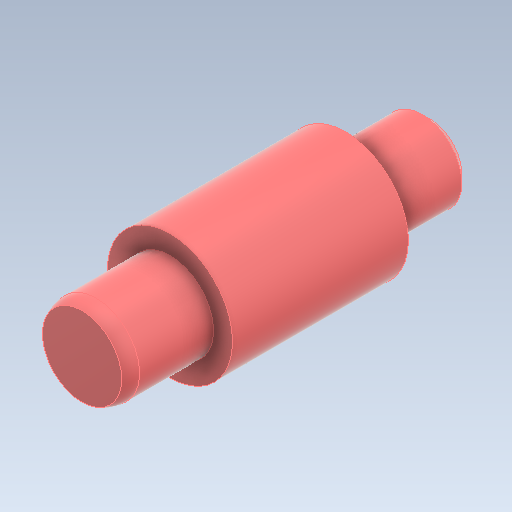
# Autodesk Inventor part: shaft
Saved by Autodesk Inventor 2021 (Build 250183000, 183)
## iProperties
Created: 2022-04-30
Part Number: shaft
Material: Generic
Document SubType Name: Modeling
Designer: authe
Density: 1 g/cm^3
Appearance: Smooth - Red
Author: authe
Autodesk Inventor part; units mm, degrees
ref_plane "YZ Plane" through (0, 0, 0) normal (1, 0, 0) x (0, 1, 0)
ref_plane "XZ Plane" through (0, 0, 0) normal (0, 1, 0) x (-1, 0, 0)
ref_plane "XY Plane" through (0, 0, 0) normal (0, 0, 1) x (1, 0, 0)
sketch "Sketch1" plane through (0, 0, 0) normal (1, 0, 0) x (0, 1, 0)
  line L0 (30.4706, 7.3849) -> (30.4706, 41.1619)
  line L1 (25.6011, 41.1619) -> (24.6173, 41.1619)
  line L2 (25.6011, 62.6619) -> (25.6011, 41.1619)
  line L3 (14.4706, 63.6457) -> (24.6173, 63.6457)
  line L4 (25.6011, 62.6619) -> (24.6173, 63.6457)
  line L5 (25.6011, -3.8381) -> (24.6173, -3.8381)
  line L6 (30.4706, 7.3849) -> (30.4706, -3.8381)
  line L7 (30.4706, 41.1619) -> (25.6011, 41.1619)
  line L8 (30.4706, -3.8381) -> (25.6011, -3.8381)
  line L9 (14.4706, 71.7924) -> (14.4706, 14.0111)
  line L10 (24.6173, -3.8381) -> (24.6173, -23.3381)
  line L11 (22.6173, -25.3381) -> (14.4706, -25.3381)
  line L12 (14.4706, -25.3381) -> (14.4706, 14.0111)
  line L13 (24.6173, -23.3381) -> (22.6173, -25.3381)
  point P0 (24.6173, -25.3381)
  point P1 (14.4706, 63.6457)
  dimension "d26" = 45
  dimension "d27" = 21.5
  dimension "d28" = 21.5
  dimension "d29" = 2
  dimension "d30" = 2
  constraints: 28 end point, 3 point on line, 2 horizontal, 1 collinear, 1 perpendicular, 1 vertical
  measures "d26" distance of L6.end L7.start
  measures "d27" distance of L2.start L2.end
  measures "d28" distance of L5.end point (24.617, -25.338)
  measures "d29" distance of L10.end point (24.617, -25.338)
  measures "d30" distance of L11.start point (24.617, -25.338)
revolve "Revolution1" add sketch "Sketch1" angle 360 about axis through (0, 14.4706, 71.7924) along (0, 0, -1)
fillet "Fillet1" radius 7 1 edges at (0, 3.3402, 62.6619)
equation "\"d30\" = d29"
body "Solid1"
